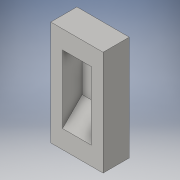
# Autodesk Inventor part: rod_socket
Saved by Autodesk Inventor 2016 (Build 200138000, 138)
## iProperties
Created: 2016-01-30
Part Number: rod_socket
Material: Generic
Document SubType Name: Modeling
Designer: Greg
Density: 1 g/cm^3
Appearance: Default
Author: Greg
Autodesk Inventor part; units mm, degrees
ref_plane "YZ Plane" through (0, 0, 0) normal (1, 0, 0) x (0, 1, 0)
ref_plane "XZ Plane" through (0, 0, 0) normal (0, 1, 0) x (-1, 0, 0)
ref_plane "XY Plane" through (0, 0, 0) normal (0, 0, 1) x (1, 0, 0)
sketch "Sketch1" plane through (0, 0, 0) normal (0, 0, 1) x (1, 0, 0)
  line L0 (-20, 40) -> (20, 40)
  line L1 (20, 40) -> (20, -40)
  line L2 (20, -40) -> (-20, -40)
  line L3 (-20, -40) -> (-20, 40)
  line L4 (0, 0) -> (10, 0) construction
  line L5 (0, 0) -> (0, -10) construction
  dimension "d0" = 40
  dimension "d1" = 80
  dimension "d2" = 10
  dimension "d3" = 10
  constraints: 12 end point, 2 horizontal, 2 parallel, 1 perpendicular, 1 vertical, 2 other
  measures "d0" distance of L1.end L2.end
  measures "d1" distance of L0.end L1.end
  measures "d2" distance of L4.start L4.end
  measures "d3" distance of L4.start L5.end
extrude "Extrusion1" add sketch "Sketch1" along normal blind 20
sketch "Sketch2" plane through (0, 0, 20) normal (0, 0, 1) x (1, 0, 0)
  line L0 (0, 0) -> (0, 10) construction
  line L1 (0, 0) -> (10, 0) construction
  line L2 (-11, 11) -> (11, 11)
  line L3 (11, 11) -> (11, -11)
  line L4 (11, -11) -> (-11, -11)
  line L5 (-11, -11) -> (-11, 11)
  dimension "d6" = 10
  dimension "d7" = 10
  dimension "d8" = 22
  dimension "d9" = 22
  constraints: 12 end point, 2 horizontal, 2 parallel, 1 perpendicular, 1 vertical, 2 other
  measures "d6" distance of L0.start L0.end
  measures "d7" distance of L0.start L1.end
  measures "d8" distance of L3.end L4.end
  measures "d9" distance of L2.end L3.end
extrude "Extrusion2" cut sketch "Sketch2" against normal blind 15
chamfer "Chamfer1" distance 15 angle 45 1 edges at (0, -11, 20)
chamfer "Chamfer2" distance 15 angle 45 1 edges at (0, 11, 20)
body "Solid1"
